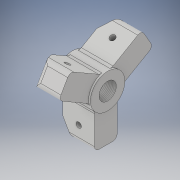
# Autodesk Inventor part: aranha
Saved by Autodesk Inventor 2017 (Build 210142000, 142)
## iProperties
Created: 2019-10-09
Part Number: aranha
Material: Generic
Document SubType Name: Modeling
Designer: 20171enpro0154
Density: 1 g/cm^3
Appearance: Default
Author: 20171enpro0154
Autodesk Inventor part; units mm, degrees
ref_plane "YZ Plane" through (0, 0, 0) normal (1, 0, 0) x (0, 1, 0)
ref_plane "XZ Plane" through (0, 0, 0) normal (0, 1, 0) x (-1, 0, 0)
sketch "Sketch1" plane through (0, 0, 0) normal (1, 0, 0) x (0, 1, 0)
  circle A0 centre (0, 0) radius 19
  circle A1 centre (0, 0) radius 9.525
  dimension "d0" = 38
  dimension "d1" = 19.05
  constraints: 2 centre point, 2 coincident
  measures "d0" diameter of A0
  measures "d1" diameter of A1
extrude "Extrusion1" add sketch "Sketch1" along normal blind 39
ref_plane "Work Plane1" through (2, 0, 0) normal (-1, 0, 0) x (0, 0, 1)
sketch "Sketch3" plane through (2, 0, 0) normal (-1, 0, 0) x (0, 0, 1)
  line L0 (0, 0) -> (-53, 0) construction
  line L1 (-48, 12.5) -> (-14.3091, 12.5)
  line L2 (-48, -12.5) -> (-14.3091, -12.5)
  circle A0 centre (0, 0) radius 19 projected
  line L3 (-48, 12.5) -> (-53, 12.5)
  line L4 (-53, -12.5) -> (-48, -12.5)
  line L5 (-53, 12.5) -> (-53, -12.5)
  dimension "d14" = 25
  constraints: 12 end point, 4 horizontal, 2 point on circle, 1 parallel, 1 point on line, 1 vertical
  measures "d14" distance of L3.end L4.start
extrude "Extrusion2" add sketch "Sketch3" against normal blind 35 contours L1 A0 L2 L4 L5 L3
sketch "Sketch4" plane through (2, -12.5, -48) normal (0, -1, 0) x (1, 0, 0)
  line L0 (-9.6665, 48) -> (46.4461, 48) construction
  line L1 (0, -5) -> (35, -5) projected
  circle A0 centre (17.5, 12) radius 3
  line L2 (17.5, 12) -> (-11.0793, 12) construction
  line L3 (0, 33.6909) -> (0, -5) projected
  line L4 (0, 12) -> (9.815, -5)
  line L5 (0, 12) -> (29, 12) construction
  line L6 (9.815, -5) -> (0, -5)
  line L7 (0, 12) -> (0, -5)
  point P0 (-2, 48)
  point P1 (0, 0)
  dimension "d19" = 6
  dimension "d22" = 60
  constraints: 12 end point, 3 horizontal, 3 point on line, 2 collinear, 1 centre point
  measures "d19" diameter of A0
  measures "d22" angle of L4 L5
extrude "Extrusion3" cut sketch "Sketch4" against normal blind 25
fillet "Fillet1" radius 5 5 edges at (11.815, 0, -53) (24.4075, 12.5, -53) (24.4075, -12.5, -53) (19.5, -12.5, -14.3091) (19.5, 12.5, -14.3091)
fillet "Fillet2" radius 3 1 edges at (2, 0, -36)
pattern_circular "Circular Pattern1" count 3 over 360 about axis through (0, 0, 0) along (1, 0, 0) of "Extrusion2", "Extrusion3", "Fillet1", "Fillet2"
thread "Thread1" size "M20x1.5" class "6H" standard "ANSI Metric M Profile" full length
body "Solid1"
